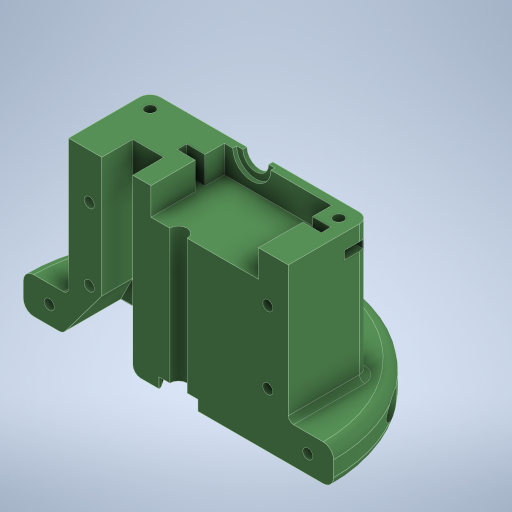
# Autodesk Inventor part: Base_1R
Saved by Autodesk Inventor 2023 (Build 270158000, 158)
## iProperties
Created: 2024-07-30
Part Number: Base_1R
Material: Generic
Document SubType Name: Modeling
Designer: Swoby
Density: 1 g/cm^3
Appearance: Default
Author: Swoby
Autodesk Inventor part; units mm, degrees
ref_plane "YZ Plane" through (0, 0, 0) normal (1, 0, 0) x (0, 1, 0)
sketch "Sketch1" plane through (0, 0, 0) normal (0, 0, 1) x (1, 0, 0)
  arc A0 (-42.5, 0) -> (42.5, 0) centre (0, 0) ccw
  line L0 (-42.5, 0) -> (-42.5, -52.5)
  line L1 (-42.5, -52.5) -> (42.5, -52.5)
  line L2 (42.5, -52.5) -> (42.5, 0)
  line L3 (-42.5, 0) -> (42.5, 0)
  arc A1 (42.5, 0) -> (-42.5, 0) centre (0, 0) ccw construction
  dimension "d0" = 85
  dimension "d1" = 52.5
  constraints: 8 end point, 4 point on circle, 3 perpendicular, 2 centre point, 2 tangent, 1 coincident, 1 vertical
  measures "d0" diameter of A0
  measures "d1" distance from line of L1 point (0, 0)
extrude "Extrusion1" add sketch "Sketch1" along normal blind 31.5
sketch "Sketch2" plane through (-42.5, 0, 0) normal (0, 1, 0) x (1, 0, 0)
  line L0 (31.85, -43.7) -> (73.45, -43.7)
  line L1 (73.45, -3.1) -> (31.85, -3.1)
  line L2 (35.1, -3.1) -> (49.9, -3.1)
  line L3 (49.9, -3.1) -> (49.9, -1.6)
  line L4 (49.9, -1.6) -> (35.1, -1.6)
  line L5 (35.1, -1.6) -> (35.1, -3.1)
  line L6 (37.5, -1.6) -> (47.5, -1.6)
  line L7 (47.5, -1.6) -> (47.5, 0)
  line L8 (47.5, 0) -> (37.5, 0)
  line L9 (37.5, 0) -> (37.5, -1.6)
  line L10 (85, 0) -> (0, 0) projected
  line L11 (31.85, -10.6) -> (24.75, -10.6)
  line L12 (24.75, -10.6) -> (24.75, -14.3)
  line L13 (24.75, -14.3) -> (31.85, -14.3)
  line L14 (73.45, -14.3) -> (80.55, -14.3)
  line L15 (80.55, -14.3) -> (80.55, -10.6)
  line L16 (80.55, -10.6) -> (73.45, -10.6)
  line L17 (31.85, -3.1) -> (31.85, -10.6)
  line L18 (73.45, -43.7) -> (73.45, -14.3)
  line L19 (73.45, -10.6) -> (73.45, -3.1)
  line L20 (31.85, -39.8) -> (25.85, -39.8)
  line L21 (25.85, -39.8) -> (25.85, -34.4)
  line L22 (25.85, -34.4) -> (31.85, -34.4)
  line L23 (31.85, -34.4) -> (31.85, -39.8) construction
  line L24 (31.85, -14.3) -> (31.85, -34.4)
  line L25 (31.85, -39.8) -> (31.85, -43.7)
  point P0 (42.5, 0)
  point P1 (49.9, -2.35)
  point P2 (42.5, -1.6)
  point P3 (42.5, -3.1)
  point P4 (42.5, 0)
  dimension "d4" = 14.8
  dimension "d5" = 1.5
  dimension "d6" = 10
  dimension "d7" = 1.6
  dimension "d9" = 41.6
  dimension "d10" = 40.6
  dimension "d11" = 7.5
  dimension "d12" = 3.7
  dimension "d13" = 7.1
  dimension "d14" = 7.1
  dimension "d15" = 10.65
  dimension "d16" = 3.9
  dimension "d17" = 5.4
  dimension "d18" = 6
  constraints: 50 end point, 15 parallel, 7 perpendicular, 6 horizontal, 6 midpoint, 4 point on line, 3 collinear
  measures "d4" distance from line of point (49.9, -2.35) L5
  measures "d5" distance of L2.end L3.end
  measures "d6" distance between parallel lines of L7 L9
  measures "d7" distance of L6.end L7.end
  measures "d9" distance of L1.start L1.end
  measures "d10" distance of L0.end L1.start
  measures "d11" distance of L1.end L11.start
  measures "d12" distance of L11.end L12.end
  measures "d13" distance of L11.start L11.end
  measures "d14" distance of L15.end L16.end
  measures "d15" distance from line of L17 point (42.5, -3.1)
  measures "d16" distance between parallel lines of L0 L20
  measures "d17" distance of L20.end L21.end
  measures "d18" distance of L21.end L22.end
extrude "Extrusion2" cut sketch "Sketch2" against normal blind 10.6 contours L25 L20 L21 L22 L24 L13 L12 L11 L17 L1 L19 L16 L15 L14 L18 L0
sketch "Sketch3" plane through (-42.5, 0, 0) normal (0, 1, 0) x (1, 0, 0)
  line L0 (31.85, -31.5) -> (31.85, -14.3) projected
  line L1 (31.85, -14.3) -> (24.75, -14.3) projected
  line L2 (24.75, -14.3) -> (24.75, -10.6) projected
  line L3 (24.75, -10.6) -> (31.85, -10.6) projected
  line L4 (31.85, -10.6) -> (31.85, -3.1) projected
  line L5 (31.85, -3.1) -> (73.45, -3.1) projected
  line L6 (73.45, -3.1) -> (73.45, -10.6) projected
  line L7 (73.45, -10.6) -> (80.55, -10.6) projected
  line L8 (80.55, -10.6) -> (80.55, -14.3) projected
  line L9 (80.55, -14.3) -> (73.45, -14.3) projected
  line L10 (73.45, -14.3) -> (73.45, -31.5) projected
  line L11 (85, -31.5) -> (73.45, -31.5) projected
  line L12 (85, 0) -> (85, -31.5) projected
  line L13 (85, 0) -> (0, 0) projected
  line L14 (0, 0) -> (0, -31.5) projected
  line L15 (31.85, -31.5) -> (0, -31.5) projected
  line L16 (42.5, -3.1) -> (42.5, 0)
  line L17 (42.5, 0) -> (47.5, 0)
  line L18 (47.5, 0) -> (47.5, -1.6)
  line L19 (47.5, -1.6) -> (49.9, -1.6)
  line L20 (49.9, -1.6) -> (49.9, -3.1)
  line L21 (49.9, -3.1) -> (42.5, -3.1)
  point P0 (49.9, -2.35)
  dimension "d21" = 5
  dimension "d22" = 1.6
  dimension "d23" = 1.5
  dimension "d24" = 7.4
  constraints: 12 end point, 3 point on line, 2 perpendicular, 1 collinear, 1 midpoint, 1 vertical
  measures "d21" distance of L16.end L17.end
  measures "d22" distance of L17.end L18.end
  measures "d23" distance of L19.end L20.end
  measures "d24" distance from line of point (49.9, -2.35) L16
revolve "Revolution1" cut sketch "Sketch3" angle 360 about axis through (0, 0, 3.1) along (0, 0, -1) contours L13 L18 L19 L20 L5 L16
sketch "Sketch4" plane through (-42.5, -52.5, 0) normal (0, -1, 0) x (1, 0, 0)
  line L0 (0, 31.5) -> (85, 31.5) projected
  arc A0 (-17.5, 31.5) -> (102.5, 31.5) centre (42.5, 31.5) ccw
  line L1 (102.5, 31.5) -> (-17.5, 31.5)
  arc A1 (102.5, 31.5) -> (-17.5, 31.5) centre (42.5, 31.5) ccw construction
  point P0 (42.5, 0)
  dimension "d26" = 120
  constraints: 4 point on circle, 3 midpoint, 2 centre point, 2 end point, 1 horizontal
  measures "d26" diameter of A0
extrude "Extrusion3" add sketch "Sketch4" along normal blind 14
sketch "Sketch5" plane through (0, 0, 31.5) normal (0, 0, 1) x (1, 0, 0)
  line L0 (-34.5, -17.6) -> (34.5, -17.6) construction
  line L1 (34.5, -17.6) -> (34.5, -45.5) construction
  line L2 (34.5, -45.5) -> (-34.5, -45.5) construction
  line L3 (-34.5, -45.5) -> (-34.5, -17.6) construction
  line L4 (-42.5, -52.5) -> (-60, -52.5) projected
  line L5 (30.95, -10.6) -> (-10.65, -10.6) projected
  line L6 (-42.5, 0) -> (-42.5, -52.5) projected
  line L7 (42.5, -52.5) -> (42.5, 0) projected
  circle A0 centre (-34.5, -17.6) radius 2
  circle A1 centre (-34.5, -45.5) radius 2
  circle A2 centre (34.5, -45.5) radius 2
  circle A3 centre (34.5, -17.6) radius 2
  line L8 (-60, -52.5) -> (-60, -66.5) projected
  line L9 (60, -66.5) -> (-60, -66.5) projected
  line L10 (60, -52.5) -> (60, -66.5) projected
  line L11 (60, -52.5) -> (42.5, -52.5) projected
  line L12 (-10.65, 0) -> (-42.5, 0) projected
  line L13 (42.5, 0) -> (30.95, 0) projected
  line L14 (-10.65, -10.6) -> (-10.65, 0) projected
  line L15 (30.95, 0) -> (30.95, -10.6) projected
  line L16 (-60, -59.5) -> (60, -59.5) construction
  circle A4 centre (-50, -59.5) radius 2
  circle A5 centre (50, -59.5) radius 2
  point P0 (0, 0)
  dimension "d29" = 7
  dimension "d30" = 7
  dimension "d31" = 8
  dimension "d32" = 8
  dimension "d33" = 4
  dimension "d34" = 4
  dimension "d35" = 4
  dimension "d36" = 4
  dimension "d71" = 4
  dimension "d72" = 4
  dimension "d73" = 10
  dimension "d74" = 10
  constraints: 10 end point, 6 centre point, 4 coincident, 2 midpoint, 2 parallel, 2 point on line, 1 horizontal, 1 perpendicular
  measures "d29" distance between parallel lines of L4 L2
  measures "d30" distance between parallel lines of L5 L0
  measures "d31" distance between parallel lines of L6 L3
  measures "d32" distance between parallel lines of L7 L1
  measures "d33" diameter of A0
  measures "d34" diameter of A1
  measures "d35" diameter of A2
  measures "d36" diameter of A3
  measures "d71" diameter of A4
  measures "d72" diameter of A5
  measures "d73" distance from line of L8 A4.centre
  measures "d74" distance from line of L10 A5.centre
extrude "Extrusion4" cut sketch "Sketch5" against normal through all contours A0 | A1 | A2 | A3 | A4 | A5
ref_plane "Work Plane1" through (0, 0, 25.5) normal (0, 0, 1) x (1, 0, 0)
sketch "Sketch6" plane through (0, 0, 25.5) normal (0, 0, 1) x (1, 0, 0)
  circle A0 centre (-34.5, -17.6) radius 2 projected
  circle A1 centre (-34.5, -45.5) radius 2 projected
  circle A2 centre (34.5, -17.6) radius 2 projected
  circle A3 centre (34.5, -45.5) radius 2 projected
  circle A4 centre (-34.5, -17.6) radius 3.75
  circle A5 centre (34.5, -17.6) radius 3.75
  circle A6 centre (-34.5, -45.5) radius 3.75
  circle A7 centre (34.5, -45.5) radius 3.75
  circle A8 centre (-50, -59.5) radius 2 projected
  circle A9 centre (50, -59.5) radius 2 projected
  circle A10 centre (-50, -59.5) radius 3.75
  circle A11 centre (50, -59.5) radius 3.75
  point P0 (0, 0)
  dimension "d40" = 7.5
  dimension "d41" = 7.5
  dimension "d42" = 7.5
  dimension "d43" = 7.5
  dimension "d75" = 7.5
  dimension "d76" = 7.5
  constraints: 6 centre point, 6 coincident, 2 other
  measures "d40" diameter of A4
  measures "d41" diameter of A5
  measures "d42" diameter of A6
  measures "d43" diameter of A7
  measures "d75" diameter of A10
  measures "d76" diameter of A11
extrude "Extrusion5" cut sketch "Sketch6" against normal through all contours A0 | A1 | A2 | A3 | A4 | A5 | A6 | A7 | A8 | A9 | A10 | A11
sketch "Sketch7" plane through (-42.5, 0, 31.5) normal (0, 1, 0) x (1, 0, 0)
  line L0 (49.9, 29.9) -> (49.9, 28.4) projected
  line L1 (49.9, 28.4) -> (73.45, 28.4) projected
  line L2 (73.45, 28.4) -> (73.45, 20.9) projected
  line L3 (73.45, 20.9) -> (80.55, 20.9) projected
  line L4 (80.55, 20.9) -> (80.55, 17.2) projected
  line L5 (80.55, 17.2) -> (73.45, 17.2) projected
  line L6 (73.45, 17.2) -> (73.45, 0) projected
  line L7 (85, 0) -> (73.45, 0) projected
  line L8 (85, 31.5) -> (85, 0) projected
  line L9 (85, 31.5) -> (47.5, 31.5) projected
  line L10 (47.5, 31.5) -> (47.5, 29.9) projected
  line L11 (47.5, 29.9) -> (49.9, 29.9) projected
  line L12 (35.1, 28.4) -> (35.1, 29.9) projected
  line L13 (35.1, 29.9) -> (37.5, 29.9) projected
  line L14 (37.5, 29.9) -> (37.5, 31.5) projected
  line L15 (37.5, 31.5) -> (0, 31.5) projected
  line L16 (0, 31.5) -> (0, 0) projected
  line L17 (31.85, 0) -> (0, 0) projected
  line L18 (31.85, 0) -> (31.85, 17.2) projected
  line L19 (31.85, 17.2) -> (24.75, 17.2) projected
  line L20 (24.75, 17.2) -> (24.75, 20.9) projected
  line L21 (24.75, 20.9) -> (31.85, 20.9) projected
  line L22 (31.85, 20.9) -> (31.85, 28.4) projected
  line L23 (31.85, 28.4) -> (35.1, 28.4) projected
  circle A0 centre (6, 25.5) radius 2
  circle A1 centre (6, 6) radius 2 construction
  circle A2 centre (79, 25.5) radius 2
  circle A3 centre (79, 6) radius 2 construction
  point P0 (42.5, 31.5)
  dimension "d46" = 4
  dimension "d47" = 4
  dimension "d48" = 4
  dimension "d49" = 4
  dimension "d50" = 6
  dimension "d51" = 6
  dimension "d52" = 6
  dimension "d53" = 6
  dimension "d54" = 6
  dimension "d55" = 6
  dimension "d56" = 6
  dimension "d57" = 6
  constraints: 4 centre point
  measures "d46" diameter of A0
  measures "d47" diameter of A1
  measures "d48" diameter of A2
  measures "d49" diameter of A3
  measures "d50" distance from line of L9 A2.centre
  measures "d51" distance from line of L8 A2.centre
  measures "d52" distance from line of L7 A3.centre
  measures "d53" distance from line of L8 A3.centre
  measures "d54" distance from line of L15 A0.centre
  measures "d55" distance from line of L16 A0.centre
  measures "d56" distance from line of L17 A1.centre
  measures "d57" distance from line of L16 A1.centre
extrude "Extrusion6" cut sketch "Sketch7" against normal blind 10 contours A0 | A2
ref_plane "Work Plane2" through (42.5, -6, 31.5) normal (0, 1, 0) x (1, 0, 0)
sketch "Sketch8" plane through (42.5, -6, 31.5) normal (0, 1, 0) x (1, 0, 0)
  circle A0 centre (-6, 25.5) radius 2 construction
  circle A1 centre (-79, 25.5) radius 2 construction
  line L0 (-8.9, 27.1743) -> (-6, 28.8486) construction
  line L1 (-6, 28.8486) -> (-3.1, 27.1743) construction
  line L2 (-3.1, 27.1743) -> (-3.1, 23.8257) construction
  line L3 (-3.1, 23.8257) -> (-6, 22.1514) construction
  line L4 (-6, 22.1514) -> (-8.9, 23.8257) construction
  line L5 (-8.9, 23.8257) -> (-8.9, 27.1743) construction
  line L6 (-76.1, 23.8257) -> (-79, 22.1514) construction
  line L7 (-79, 22.1514) -> (-81.9, 23.8257) construction
  line L8 (-81.9, 23.8257) -> (-81.9, 27.1743) construction
  line L9 (-81.9, 27.1743) -> (-79, 28.8486) construction
  line L10 (-79, 28.8486) -> (-76.1, 27.1743) construction
  line L11 (-76.1, 27.1743) -> (-76.1, 23.8257) construction
  line L12 (-11.55, 17.2) -> (-11.55, 0) construction
  line L13 (-11.55, 28.4) -> (-11.55, 20.9) construction
  line L14 (-9.2, 27.3475) -> (-6, 29.195)
  line L15 (-6, 29.195) -> (-2.8, 27.3475)
  line L16 (-2.8, 27.3475) -> (-2.8, 23.6525)
  line L17 (-2.8, 23.6525) -> (-6, 21.805)
  line L18 (-6, 21.805) -> (-9.2, 23.6525)
  line L19 (-9.2, 23.6525) -> (-9.2, 27.3475)
  line L20 (-75.8, 27.3475) -> (-79, 29.195)
  line L21 (-79, 29.195) -> (-82.2, 27.3475)
  line L22 (-82.2, 27.3475) -> (-82.2, 23.6525)
  line L23 (-82.2, 23.6525) -> (-79, 21.805)
  line L24 (-79, 21.805) -> (-75.8, 23.6525)
  line L25 (-75.8, 23.6525) -> (-75.8, 27.3475)
  line L26 (17.5, 0) -> (-102.5, 0) projected
  arc A2 (17.5, 0) -> (-102.5, 0) centre (-42.5, 0) ccw projected
  line L27 (-11.75, 31.5) -> (-4.25, 31.5) projected
  line L28 (-80.75, 31.5) -> (-73.25, 31.5) projected
  line L29 (-11.75, 31.5) -> (-4.25, 31.5) projected
  line L30 (-80.75, 31.5) -> (-73.25, 31.5) projected
  line L31 (-47.5, 31.5) -> (-37.5, 31.5) projected
  line L32 (0, 31.5) -> (-37.5, 31.5) projected
  line L33 (-85, 31.5) -> (0, 31.5) projected
  line L34 (-47.5, 31.5) -> (-85, 31.5) projected
  line L35 (-85, 31.5) -> (-85, 0) projected
  line L36 (-85, 31.5) -> (-85, 0) projected
  line L37 (0, 31.5) -> (0, 0) projected
  line L38 (0, 31.5) -> (0, 0) projected
  line L39 (-6, 0) -> (-10, 0) projected
  line L40 (-75, 0) -> (-79, 0) projected
  line L41 (-6, 0) -> (-10, 0) projected
  line L42 (-75, 0) -> (-79, 0) projected
  line L43 (-53.15, 0) -> (-85, 0) projected
  line L44 (-85, 0) -> (-102.5, 0) projected
  line L45 (17.5, 0) -> (-102.5, 0) projected
  line L46 (17.5, 0) -> (0, 0) projected
  line L47 (0, 0) -> (-11.55, 0) projected
  line L48 (-11.55, 0) -> (-53.15, 0) projected
  line L49 (-6, 21.805) -> (0, 21.805)
  line L50 (-6, 29.195) -> (0, 29.195)
  line L51 (0, 21.805) -> (0, 29.195)
  line L52 (-79, 29.195) -> (-85, 29.195)
  line L53 (-85, 29.195) -> (-85, 21.805)
  line L54 (-79, 21.805) -> (-85, 21.805)
  point P0 (-42.5, 31.5)
  point P1 (-85, 29.195)
  point P2 (-85, 21.805)
  point P3 (0, 21.805)
  point P4 (0, 29.195)
  dimension "d64" = 0.3
  dimension "d65" = 0.3
  dimension "d69" = 5.8
  dimension "d70" = 5.8
  dimension "d91" = 6.4
  constraints: 60 end point, 6 point on line, 3 parallel, 2 coincident, 1 perpendicular, 36 other
  measures "d64" distance between parallel lines of L5 L19
  measures "d65" distance between parallel lines of L10 L20
  measures "d69" distance between parallel lines of L5 L2
  measures "d70" distance between parallel lines of L8 L11
  measures "d91" distance between parallel lines of L19 L16
extrude "Extrusion7" cut sketch "Sketch8" against normal blind 3.3 contours L14 L15 L16 L17 L18 L19 | L50 L37 L49 L17 L16 L15 | L35 L52 L21 L22 L23 L54 | L23 L22 L21 L20 L25 L24
fillet "Fillet1" radius 4 4 edges at (0, -52.5, -28.5) (42.5, -26.25, 0) (-42.5, -26.25, 0) (0, -66.5, -28.5)
sketch "Sketch9" plane through (-42.5, 0, 31.5) normal (0, 1, 0) x (1, 0, 0)
  line L0 (24.85, 0) -> (12.85, 0)
  line L1 (12.85, 0) -> (12.85, 12)
  line L2 (12.85, 12) -> (24.85, 12)
  line L3 (24.85, 12) -> (24.85, 0)
  line L4 (-5.5, 0) -> (-9.5, 0) projected
  line L5 (79, 0) -> (75, 0) projected
  line L6 (10, 0) -> (6, 0) projected
  line L7 (94.5, 0) -> (90.5, 0) projected
  line L8 (79, 0) -> (75, 0) projected
  line L9 (10, 0) -> (6, 0) projected
  line L10 (98.5, 0) -> (102.5, 0) projected
  line L11 (98.5, 0) -> (85, 0) projected
  line L12 (85, 0) -> (73.45, 0) projected
  line L13 (73.45, 0) -> (31.85, 0) projected
  line L14 (31.85, 0) -> (0, 0) projected
  line L15 (0, 0) -> (-13.5, 0) projected
  line L16 (-17.5, 0) -> (-13.5, 0) projected
  line L17 (98.5, 0) -> (-13.5, 0) projected
  line L18 (0, 27.5) -> (0, 0) projected
  line L19 (0, 27.5) -> (0, 0) projected
  line L20 (0, 27.5) -> (0, 21.805) projected
  line L21 (0, 21.805) -> (0, 27.5) projected
  line L22 (102.5, 0) -> (98.5, 0) projected
  line L23 (-13.5, 0) -> (-17.5, 0) projected
  point P0 (42.5, 31.5)
  point P1 (12.85, 6)
  dimension "d78" = 12
  dimension "d79" = 12.85
  dimension "d80" = 12
  constraints: 8 end point, 2 parallel, 1 horizontal, 1 midpoint, 1 perpendicular, 1 point on line
  measures "d78" distance of L1.end L2.end
  measures "d79" distance from line of point (12.85, 6) L19
  measures "d80" distance of L0.end L1.end
extrude "Extrusion8" cut sketch "Sketch9" against normal through all
sketch "Sketch10" plane through (0, 0, 0) normal (1, 0, 0) x (0, 1, 0)
  line L0 (-13.85, 0) -> (-21.35, 0) projected
  line L1 (-41.75, 0) -> (-49.25, 0) projected
  line L2 (-41.75, 0) -> (-49.25, 0) projected
  line L3 (-13.85, 0) -> (-21.35, 0) projected
  line L4 (0, 0) -> (-52.5, 0) projected
  line L5 (0, 0) -> (0, 0) projected
  line L6 (-52.5, 0) -> (0, 0) projected
  line L7 (-52.5, 31.5) -> (-52.5, 31.5) projected
  line L8 (-52.5, 4) -> (-52.5, 31.5) projected
  line L9 (-52.5, 0) -> (-52.5, 4) projected
  line L10 (-52.5, 4) -> (-52.5, 0) projected
  line L11 (-52.5, 4) -> (-52.5, 31.5) projected
  line L12 (-52.5, 0) -> (-32.5, 0)
  line L13 (-32.5, 0) -> (-52.5, -15)
  line L14 (-52.5, -15) -> (-52.5, 0)
  point P0 (0, 0)
  dimension "d83" = 20
  dimension "d84" = 15
  constraints: 6 end point, 1 perpendicular, 1 point on line
  measures "d83" distance of L10.end L12.end
  measures "d84" distance of L13.end L10.end
extrude "Extrusion9" add sketch "Sketch10" along normal mid plane 5
fillet "Fillet2" radius 2 12 edges at (41.3284, -52.5, 1.1716) (20.5, -52.5, 0) (42.5, -52.5, 17.75) (2.5, -52.5, -7.5) (-41.3284, -52.5, 1.1716) (-42.5, -52.5, 17.75) (-20.5, -52.5, 0) (0, -52.5, -15) (-2.5, -52.5, -7.5) (2.5, -42.5, 0) (0, -32.5, 0) (-2.5, -42.5, 0)
sketch "Sketch11" plane through (-17.75, 0, 14.3) normal (0, 1, 0) x (1, 0, 0)
  arc A0 (65.5, 19.1309) -> (-30, 19.1309) centre (17.75, -17.2) ccw projected
  arc A1 (65.5, 19.1309) -> (-30, 19.1309) centre (17.75, -17.2) ccw projected
  circle A2 centre (17.75, -17.2) radius 3.4
  point P0 (17.75, 14.3)
  dimension "d88" = 6.8
  constraints: 1 centre point, 1 coincident, 2 other
  measures "d88" diameter of A2
extrude "Extrusion10" cut sketch "Sketch11" against normal through all
sketch "Sketch12" plane through (-42.5, -66.5, 0) normal (0, -1, 0) x (1, 0, 0)
  arc A0 (39.1, 31.5) -> (45.9, 31.5) centre (42.5, 31.5) ccw projected
  arc A1 (39.1, 31.5) -> (45.9, 31.5) centre (42.5, 31.5) ccw projected
  line L0 (42.5, 31.5) -> (29.5953, 18.5953)
  line L1 (42.5, 31.5) -> (60.75, 31.5) construction
  line L2 (42.5, 31.5) -> (52.4582, 31.5) construction
  circle A2 centre (31.0095, 20.0095) radius 2
  line L3 (40.6969, 24.1107) -> (35.1107, 29.6969) construction
  line L4 (40.6969, 24.1107) -> (32.1252, 18.3496)
  line L5 (35.1107, 29.6969) -> (29.3496, 21.1252)
  line L6 (42.5, 31.5) -> (55.4047, 18.5953) construction
  circle A3 centre (53.9905, 20.0095) radius 2
  line L7 (49.8893, 29.6969) -> (44.3031, 24.1107) construction
  line L8 (49.8893, 29.6969) -> (55.6504, 21.1252)
  line L9 (44.3031, 24.1107) -> (52.8748, 18.3496)
  line L10 (42.5, 31.5) -> (55.4047, 44.4047)
  circle A4 centre (53.9905, 42.9905) radius 2
  line L11 (44.3031, 38.8893) -> (49.8893, 33.3031)
  line L12 (44.3031, 38.8893) -> (52.8748, 44.6504)
  line L13 (49.8893, 33.3031) -> (55.6504, 41.8748)
  line L14 (42.5, 31.5) -> (29.5953, 44.4047)
  circle A5 centre (31.0095, 42.9905) radius 2
  line L15 (35.1107, 33.3031) -> (40.6969, 38.8893)
  line L16 (35.1107, 33.3031) -> (29.3496, 41.8748)
  line L17 (40.6969, 38.8893) -> (32.1252, 44.6504)
  arc A6 (49.8893, 33.3031) -> (49.3396, 31.5) centre (52.572, 31.5) ccw
  arc A7 (44.3031, 24.1107) -> (40.6969, 24.1107) centre (42.5, 21.428) ccw
  arc A8 (49.3396, 31.5) -> (49.8893, 29.6969) centre (52.572, 31.5) ccw
  arc A9 (35.1107, 29.6969) -> (35.1107, 33.3031) centre (32.428, 31.5) ccw
  line L18 (49.3396, 31.5) -> (35.6604, 31.5)
  point P0 (42.5, 0)
  point P1 (37.9038, 26.9038)
  point P2 (47.0962, 26.9038)
  point P3 (47.0962, 36.0962)
  point P4 (37.9038, 36.0962)
  point P5 (45.9, 31.5)
  point P6 (35.6604, 31.5)
  dimension "d92" = 135
  dimension "d94" = 18.25
  dimension "d95" = 4
  dimension "d96" = 6.5
  dimension "d97" = 7.9
  dimension "d100" = 360
  constraints: 38 end point, 21 point on circle, 9 point on line, 9 tangent, 8 centre point, 2 horizontal, 1 equal length, 1 midpoint, 1 perpendicular, 53 other
  measures "d92" angle of L0 L1
  measures "d94" distance of L0.start L0.end
  measures "d95" diameter of A2
  measures "d96" distance from line of A0.centre L3
  measures "d97" distance of L3.start L3.end
extrude "Extrusion11" cut sketch "Sketch12" against normal blind 4 contours A0 L0 A2 L5 A9 L18 | A0 L18 A8 L8 A3 L9 A7 L4 A2 L0 | A2 L0 | L0 A2 | A3
sketch "Sketch13" plane through (-42.5, -66.5, 0) normal (0, -1, 0) x (1, 0, 0)
  line L0 (45.9, 31.5) -> (49.3396, 31.5) projected
  arc A0 (39.1, 31.5) -> (45.9, 31.5) centre (42.5, 31.5) ccw projected
  line L1 (35.6604, 31.5) -> (39.1, 31.5) projected
  arc A1 (35.1107, 29.6969) -> (35.6604, 31.5) centre (32.428, 31.5) ccw projected
  line L2 (29.3496, 21.1252) -> (35.1107, 29.6969) projected
  arc A2 (29.3496, 21.1252) -> (32.1252, 18.3496) centre (31.0095, 20.0095) ccw projected
  line L3 (40.6969, 24.1107) -> (32.1252, 18.3496) projected
  arc A3 (44.3031, 24.1107) -> (40.6969, 24.1107) centre (42.5, 21.428) ccw projected
  line L4 (52.8748, 18.3496) -> (44.3031, 24.1107) projected
  arc A4 (52.8748, 18.3496) -> (55.6504, 21.1252) centre (53.9905, 20.0095) ccw projected
  line L5 (49.8893, 29.6969) -> (55.6504, 21.1252) projected
  arc A5 (49.3396, 31.5) -> (49.8893, 29.6969) centre (52.572, 31.5) ccw projected
  arc A6 (43.9126, 23.5298) -> (41.0874, 23.5298) centre (42.5, 21.428) ccw
  line L6 (41.0874, 23.5298) -> (32.5156, 17.7686)
  arc A7 (28.7686, 21.5156) -> (32.5156, 17.7686) centre (31.0095, 20.0095) ccw
  line L7 (28.7686, 21.5156) -> (34.5298, 30.0874)
  arc A8 (34.5298, 30.0874) -> (34.8617, 32.2) centre (32.428, 31.5) ccw
  line L8 (34.8617, 32.2) -> (39.8923, 32.2)
  arc A9 (39.8923, 32.2) -> (45.1077, 32.2) centre (42.5, 31.5) ccw
  line L9 (45.1077, 32.2) -> (50.1383, 32.2)
  arc A10 (50.1383, 32.2) -> (50.4702, 30.0874) centre (52.572, 31.5) ccw
  line L10 (50.4702, 30.0874) -> (56.2314, 21.5156)
  arc A11 (52.4844, 17.7686) -> (56.2314, 21.5156) centre (53.9905, 20.0095) ccw
  line L11 (52.4844, 17.7686) -> (43.9126, 23.5298)
  point P0 (42.5, 0)
  dimension "d104" = 0.7
  constraints: 12 end point, 12 point on circle, 6 centre point, 11 other
  measures "d104" distance between parallel lines of L4 L11
extrude "Extrusion12" cut sketch "Sketch13" against normal blind 4 contours L0 A5 L5 A4 L4 A3 L3 A2 L2 A1 L1 A0 | A6 L6 A7 L7 A8 L8 A9 L9 A10 L10 A11 L11
sketch "Sketch14" plane through (-42.5, -62.5, 0) normal (0, -1, 0) x (1, 0, 0)
  arc A0 (52.4844, 17.7686) -> (56.2314, 21.5156) centre (53.9905, 20.0095) ccw projected
  arc A1 (28.7686, 21.5156) -> (32.5156, 17.7686) centre (31.0095, 20.0095) ccw projected
  circle A2 centre (53.9905, 20.0095) radius 0.5
  circle A3 centre (31.0095, 20.0095) radius 0.5
  point P0 (42.5, 0)
  dimension "d107" = 1
  dimension "d108" = 1
  constraints: 2 centre point, 2 coincident
  measures "d107" diameter of A2
  measures "d108" diameter of A3
extrude "Extrusion13" cut sketch "Sketch14" against normal blind 4
chamfer "Chamfer1" distance 15 distance2 20 1 edges at (-29.65, -66.5, 25.5) measured on face at (1.7223, -66.5, 3.5694)
chamfer "Chamfer2" distance 10 distance2 20 1 edges at (-23.65, -66.5, 19.5) measured on face at (1.7223, -66.5, 3.5694)
fillet "Fillet3" radius 3 3 edges at (-44.65, -66.5, 25.5) (-23.65, -66.5, 9.5) (-17.65, -66.5, 25.5)
equation "\"d14\" = d13"
equation "\"d70\" = d69"
body "Solid1"
